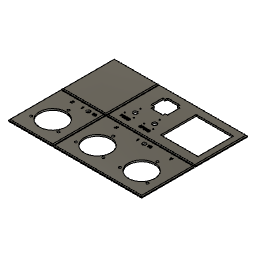
cnc3018_ctrl v79 (Autodesk Fusion 360 design; units mm, degrees)
Autodesk Fusion 360 part; units mm, degrees
sketch "panel" plane through (0, 0, 0) normal (0, 0, 1) x (1, 0, 0)
  line L0 (0, 0) -> (71, 0)
  line L1 (71, 0) -> (71, 84.5)
  line L2 (71, 84.5) -> (0, 84.5)
  line L3 (0, 84.5) -> (0, 0)
  line L4 (35.5, 84.5) -> (35.5, 0) construction
  circle A0 centre (35.5, 35.5) radius 30.5 construction
  line L5 (35.5, 66) -> (71, 66) construction
  line L6 (46.5, 79.5) -> (59.5, 79.5) construction
  line L7 (59.5, 79.5) -> (59.5, 71) construction
  line L8 (59.5, 71) -> (46.5, 71) construction
  line L9 (46.5, 71) -> (46.5, 79.5) construction
  line L10 (46.5, 79.5) -> (59.5, 71) construction
  circle A1 centre (53, 75.25) radius 3
  line L11 (66, 79.5) -> (40, 79.5) construction
  line L12 (40, 79.5) -> (40, 71) construction
  line L13 (40, 71) -> (66, 71) construction
  line L14 (66, 71) -> (66, 79.5) construction
  line L15 (66, 79.5) -> (40, 71) construction
  line L16 (40, 79.5) -> (66, 71) construction
  line L17 (40, 71) -> (46.5, 71) construction
  line L18 (46.5, 71) -> (46.5, 79.5) construction
  line L19 (46.5, 79.5) -> (40, 79.5) construction
  line L20 (40, 79.5) -> (40, 71) construction
  line L21 (59.5, 71) -> (66, 71) construction
  line L22 (66, 71) -> (66, 79.5) construction
  line L23 (66, 79.5) -> (59.5, 79.5) construction
  line L24 (59.5, 79.5) -> (59.5, 71) construction
  line L25 (24, 79.5) -> (30.5, 79.5) construction
  line L26 (30.5, 79.5) -> (30.5, 71) construction
  line L27 (30.5, 71) -> (24, 71) construction
  line L28 (24, 71) -> (24, 79.5) construction
  line L29 (24, 71) -> (30.5, 71) construction
  line L30 (30.5, 71) -> (30.5, 79.5) construction
  line L31 (30.5, 79.5) -> (24, 79.5) construction
  line L32 (24, 79.5) -> (24, 71) construction
  circle A2 centre (35.5, 35.5) radius 21.25
  circle A3 centre (35.5, 60.9) radius 1.75
  circle A4 centre (13.503, 22.8) radius 1.75
  circle A5 centre (57.497, 22.8) radius 1.75
  line L33 (71, 0) -> (213, 0)
  line L34 (213, 0) -> (213, 84.5)
  line L35 (213, 84.5) -> (71, 84.5)
  line L36 (71, 84.5) -> (71, 0)
  line L37 (35.5, 35.5) -> (213, 35.5) construction
  line L38 (53, 75.25) -> (213, 75.25) construction
  circle A6 centre (106.5, 35.5) radius 21.25
  circle A7 centre (106.5, 35.5) radius 30.5 construction
  line L39 (106.5, 35.5) -> (106.5, 84.5) construction
  circle A8 centre (106.5, 60.9) radius 1.75
  line L40 (35.5, 60.9) -> (213, 60.9) construction
  line L41 (35.5, 14.25) -> (213, 14.25) construction
  line L42 (35.5, 5) -> (213, 5) construction
  circle A9 centre (84.503, 22.8) radius 1.75
  circle A10 centre (128.497, 22.8) radius 1.75
  circle A11 centre (177.5, 35.5) radius 21.25
  circle A12 centre (177.5, 35.5) radius 30.5 construction
  line L43 (177.5, 35.5) -> (177.5, 84.5) construction
  circle A13 centre (177.5, 60.9) radius 1.75
  circle A14 centre (155.503, 22.8) radius 1.75
  circle A15 centre (199.497, 22.8) radius 1.75
  line L44 (142, 84.5) -> (142, 0) construction
  line L45 (148.5, 71) -> (135.5, 71) construction
  line L46 (135.5, 71) -> (135.5, 79.5) construction
  line L47 (135.5, 79.5) -> (148.5, 79.5) construction
  line L48 (148.5, 79.5) -> (148.5, 71) construction
  line L49 (148.5, 71) -> (135.5, 79.5) construction
  line L50 (135.5, 71) -> (148.5, 79.5) construction
  line L51 (155, 71) -> (129, 71) construction
  line L52 (129, 71) -> (129, 79.5) construction
  line L53 (129, 79.5) -> (155, 79.5) construction
  line L54 (155, 79.5) -> (155, 71) construction
  line L55 (155, 71) -> (129, 79.5) construction
  line L56 (129, 71) -> (155, 79.5) construction
  circle A16 centre (142, 75.25) radius 3
  line L57 (40, 71) -> (46.5, 71) construction
  line L58 (46.5, 71) -> (46.5, 79.5) construction
  line L59 (46.5, 79.5) -> (40, 79.5) construction
  line L60 (40, 79.5) -> (40, 71) construction
  line L61 (129, 71) -> (135.5, 71) construction
  line L62 (135.5, 71) -> (135.5, 79.5) construction
  line L63 (135.5, 79.5) -> (129, 79.5) construction
  line L64 (129, 79.5) -> (129, 71) construction
  line L65 (148.5, 71) -> (155, 71) construction
  line L66 (155, 71) -> (155, 79.5) construction
  line L67 (155, 79.5) -> (148.5, 79.5) construction
  line L68 (148.5, 79.5) -> (148.5, 71) construction
  line L69 (101.5, 79.5) -> (95, 79.5) construction
  line L70 (95, 79.5) -> (95, 71) construction
  line L71 (95, 71) -> (101.5, 71) construction
  line L72 (101.5, 71) -> (101.5, 79.5) construction
  line L73 (101.5, 79.5) -> (95, 71) construction
  line L74 (95, 79.5) -> (101.5, 71) construction
  line L75 (95, 71) -> (101.5, 71) construction
  line L76 (101.5, 71) -> (101.5, 79.5) construction
  line L77 (101.5, 79.5) -> (95, 79.5) construction
  line L78 (95, 79.5) -> (95, 71) construction
  line L79 (189, 79.5) -> (182.5, 79.5) construction
  line L80 (182.5, 79.5) -> (182.5, 71) construction
  line L81 (182.5, 71) -> (189, 71) construction
  line L82 (189, 71) -> (189, 79.5) construction
  line L83 (189, 79.5) -> (182.5, 71) construction
  line L84 (182.5, 79.5) -> (189, 71) construction
  line L85 (182.5, 71) -> (189, 71) construction
  line L86 (189, 71) -> (189, 79.5) construction
  line L87 (189, 79.5) -> (182.5, 79.5) construction
  line L88 (182.5, 79.5) -> (182.5, 71) construction
  line L89 (0, 84.5) -> (213, 84.5)
  line L90 (213, 84.5) -> (213, 169)
  line L91 (213, 169) -> (0, 169)
  line L92 (0, 169) -> (0, 84.5)
  line L93 (143, 156.5) -> (203, 156.5)
  line L94 (203, 156.5) -> (203, 99.5)
  line L95 (203, 99.5) -> (143, 99.5)
  line L96 (143, 99.5) -> (143, 156.5)
  line L97 (93.25, 156.5) -> (120.75, 156.5)
  line L98 (120.75, 156.5) -> (120.75, 129)
  line L99 (120.75, 129) -> (93.25, 129)
  line L100 (93.25, 129) -> (93.25, 156.5)
  line L101 (93.25, 156.5) -> (97.05, 156.5)
  line L102 (97.05, 156.5) -> (97.05, 152.7)
  line L103 (97.05, 152.7) -> (93.25, 152.7)
  line L104 (93.25, 152.7) -> (93.25, 156.5)
  line L105 (120.75, 156.5) -> (116.95, 156.5)
  line L106 (116.95, 156.5) -> (116.95, 152.7)
  line L107 (116.95, 152.7) -> (120.75, 152.7)
  line L108 (120.75, 152.7) -> (120.75, 156.5)
  line L109 (93.25, 129) -> (98.25, 129)
  line L110 (98.25, 129) -> (98.25, 134)
  line L111 (98.25, 134) -> (93.25, 134)
  line L112 (93.25, 134) -> (93.25, 129)
  line L113 (120.75, 129) -> (116.95, 129)
  line L114 (116.95, 129) -> (116.95, 132.8)
  line L115 (116.95, 132.8) -> (120.75, 132.8)
  line L116 (120.75, 132.8) -> (120.75, 129)
  line L117 (71, 84.5) -> (71, 169)
  line L118 (76, 124) -> (138, 124) construction
  line L119 (138, 124) -> (138, 89.5) construction
  line L120 (138, 89.5) -> (76, 89.5) construction
  line L121 (76, 89.5) -> (76, 124) construction
  circle A17 centre (91.5, 110.25) radius 3.5
  circle A18 centre (91.5, 110.25) radius 10.5 construction
  line L122 (81, 120.75) -> (102, 120.75) construction
  line L123 (102, 120.75) -> (102, 92.75) construction
  line L124 (102, 92.75) -> (81, 92.75) construction
  line L125 (81, 92.75) -> (81, 120.75) construction
  line L126 (91.5, 110.25) -> (91.5, 120.75) construction
  line L127 (81, 92.75) -> (102, 92.75) construction
  line L128 (102, 92.75) -> (102, 99.75) construction
  line L129 (102, 99.75) -> (81, 99.75) construction
  line L130 (81, 99.75) -> (81, 92.75) construction
  line L131 (81, 92.75) -> (102, 92.75) construction
  line L132 (102, 92.75) -> (102, 99.75) construction
  line L133 (102, 99.75) -> (81, 99.75) construction
  line L134 (81, 99.75) -> (81, 92.75) construction
  line L135 (76, 124) -> (107, 124) construction
  line L136 (107, 124) -> (76, 89.5) construction
  line L137 (81, 120.75) -> (102, 92.75) construction
  line L138 (91.5, 110.25) -> (98.9246, 102.8254) construction
  line L139 (91.5, 110.25) -> (84.0754, 102.8254) construction
  circle A19 centre (91.5, 120.75) radius 0.875
  circle A20 centre (84.0754, 102.8254) radius 0.875
  circle A21 centre (98.9246, 102.8254) radius 0.875
  line L140 (107, 124) -> (138, 89.5) construction
  line L141 (143, 156.5) -> (71, 156.5) construction
  line L142 (107, 124) -> (107, 89.5) construction
  line L143 (133, 92.75) -> (112, 92.75) construction
  line L144 (112, 120.75) -> (133, 120.75) construction
  line L145 (112, 92.75) -> (133, 92.75) construction
  line L146 (112, 120.75) -> (133, 92.75) construction
  circle A22 centre (122.5, 110.25) radius 10.5 construction
  line L147 (122.5, 110.25) -> (129.9246, 102.8254) construction
  circle A23 centre (129.9246, 102.8254) radius 0.875
  line L148 (122.5, 110.25) -> (122.5, 120.75) construction
  line L149 (133, 120.75) -> (133, 92.75) construction
  line L150 (122.5, 110.25) -> (115.0754, 102.8254) construction
  line L151 (133, 99.75) -> (112, 99.75) construction
  line L152 (133, 92.75) -> (133, 99.75) construction
  circle A24 centre (122.5, 120.75) radius 0.875
  circle A25 centre (115.0754, 102.8254) radius 0.875
  line L153 (112, 99.75) -> (112, 92.75) construction
  line L154 (112, 92.75) -> (112, 120.75) construction
  circle A26 centre (122.5, 110.25) radius 3.5
  line L155 (112, 92.75) -> (133, 92.75) construction
  line L156 (133, 92.75) -> (133, 99.75) construction
  line L157 (133, 99.75) -> (112, 99.75) construction
  line L158 (112, 99.75) -> (112, 92.75) construction
  point P0 (53, 75.25)
  point P1 (142, 75.25)
  point P2 (142, 75.25)
  point P3 (98.25, 75.25)
  point P4 (185.75, 75.25)
  point P5 (107, 156.5)
  point P6 (91.5, 106.75)
  point P7 (122.5, 106.75)
  dimension "d120" = 61
  dimension "d122" = 71
  dimension "d123" = 5
  dimension "d124" = 13
  dimension "d125" = 8.5
  dimension "d126" = 6
  dimension "d127" = 26
  dimension "d128" = 8.5
  dimension "d129" = 4
  dimension "d130" = 4
  dimension "d131" = 5
  dimension "d132" = 5
  dimension "d133" = 5
  dimension "d134" = 6.5
  dimension "d135" = 8.5
  dimension "d136" = 5
  dimension "d137" = 5
  dimension "d138" = 4
  dimension "d139" = 42.5
  dimension "d140" = 3.5
  dimension "d141" = 25.4
  dimension "d144" = 360
  dimension "d145" = 142
  dimension "d149" = 5
  dimension "d150" = 3.5
  dimension "d153" = 360
  dimension "d154" = 5
  dimension "d155" = 3.5
  dimension "d157" = 360
  dimension "d158" = 13
  dimension "d159" = 8.5
  dimension "d160" = 26
  dimension "d161" = 8.5
  dimension "d162" = 6
  dimension "d163" = 4
  dimension "d164" = 4
  dimension "d165" = 4
  dimension "d166" = 6.5
  dimension "d167" = 8.5
  dimension "d168" = 5
  dimension "d169" = 4
  dimension "d170" = 6.5
  dimension "d171" = 8.5
  dimension "d172" = 5
  dimension "d173" = 4
  dimension "d184" = 84.5
  dimension "d185" = 84.5
  dimension "d186" = 60
  dimension "d187" = 57
  dimension "d188" = 10
  dimension "d189" = 15
  dimension "d190" = 27.5
  dimension "d191" = 27.5
  dimension "d192" = 3.8
  dimension "d193" = 3.8
  dimension "d194" = 3.8
  dimension "d195" = 3.8
  dimension "d196" = 5
  dimension "d197" = 5
  dimension "d198" = 3.8
  dimension "d199" = 3.8
  dimension "d200" = 12.5
  dimension "d201" = 12.5
  dimension "d203" = 5
  dimension "d204" = 5
  dimension "d205" = 5
  dimension "d206" = 5
  dimension "d207" = 7
  dimension "d208" = 21
  dimension "d209" = 21
  dimension "d212" = 28
  dimension "d213" = 4
  dimension "d214" = 135
  dimension "d215" = 135
  dimension "d216" = 1.75
  dimension "d217" = 1.75
  dimension "d218" = 1.75
  dimension "d221" = 31
  dimension "d222" = 0
  dimension "d223" = 4
  text T0 "1" font "Arial" height 4 align centre middle in box 6.5 x 8.5 at (40, 71) x (1, 0) y (0, 1) spacing 1
  text T1 "10" font "Arial" height 4 align centre middle in box 6.5 x 8.5 at (59.5, 71) x (1, 0) y (0, 1) spacing 1
  text T2 "Z" font "Arial" height 4 align centre middle in box 6.5 x 8.5 at (24, 71) x (1, 0) y (0, 1) spacing 1
  text T3 "1" font "Arial" height 4 align centre middle in box 6.5 x 8.5 at (129, 71) x (1, 0) y (0, 1) spacing 1
  text T4 "10" font "Arial" height 4 align centre middle in box 6.5 x 8.5 at (148.5, 71) x (1, 0) y (0, 1) spacing 1
  text T5 "X" font "Arial" height 4 align centre middle in box 6.5 x 8.5 at (95, 71) x (1, 0) y (0, 1) spacing 1
  text T6 "Y" font "Arial" height 4 align centre middle in box 6.5 x 8.5 at (182.5, 71) x (1, 0) y (0, 1) spacing 1
  text T7 "FEED" font "Arial" height 4 align centre middle in box 21 x 7 at (81, 92.75) x (1, 0) y (0, 1) spacing 1
  text T8 "SPIND" font "Arial" height 4 align centre middle in box 21 x 7 at (112, 92.75) x (1, 0) y (0, 1) spacing 1
  constraint horizontal L0
  constraint vertical L1
  constraint horizontal L2
  constraint vertical L3
  constraint coincident L0.start L3.end
  constraint midpoint L2 L4.start
  constraint midpoint L0 L4.end
  constraint coincident A0 L5.start
  constraint coincident L4 L5.start
  constraint coincident L1 L5.end
  constraint tangent A0 L5
  constraint perpendicular L1 L5
  constraint horizontal L6
  constraint vertical L7
  constraint horizontal L8
  constraint vertical L9
  constraint coincident L10 P0
  constraint horizontal L11
  constraint perpendicular L11 L12
  constraint parallel L11 L13
  constraint parallel L12 L14
  constraint coincident L15 P0
  constraint coincident L16 P0
  constraint coincident P0 A1.centre
  constraint midpoint L10 P0
  constraint coincident L8.end
  constraint coincident L11.end
  constraint coincident L13.end
  constraint coincident L6.end
  constraint horizontal L25
  constraint vertical L26
  constraint horizontal L27
  constraint vertical L28
  constraint coincident L26.end
  constraint coincident L25.start
  constraint concentric A0 A2
  constraint coincident L4 A3.centre
  constraint horizontal L33
  constraint vertical L34
  constraint horizontal L35
  constraint vertical L36
  constraint coincident A0.centre A2.centre
  constraint coincident L34 L37.end
  constraint perpendicular L34 L37
  constraint coincident L34 L38.end
  constraint perpendicular L34 L38
  constraint coincident L37 A6.centre
  constraint concentric A6 A7
  constraint coincident A6.centre A7.centre
  constraint coincident L35 L39.end
  constraint perpendicular L35 L39
  constraint coincident L39 A8.centre
  constraint coincident A3.centre L40.start
  constraint coincident L34 L40.end
  constraint perpendicular L34 L40
  constraint coincident A8.centre L40
  constraint coincident A2 L41.start
  constraint coincident L4 L41.start
  constraint coincident L34 L41.end
  constraint tangent A2 L41
  constraint coincident A0 L42.start
  constraint coincident L4 L42.start
  constraint coincident L34 L42.end
  constraint tangent A0 L42
  constraint tangent A7 L42
  constraint tangent A6 L41
  constraint coincident L37 A11.centre
  constraint tangent L41 A11
  constraint concentric A11 A12
  constraint tangent L42 A12
  constraint coincident A11.centre A12.centre
  constraint coincident L35 L43.end
  constraint perpendicular L35 L43
  constraint coincident L43 A13.centre
  constraint coincident L40 A13.centre
  constraint midpoint L35 L44.start
  constraint midpoint L33 L44.end
  constraint horizontal L45
  constraint perpendicular L45 L46
  constraint parallel L45 L47
  constraint parallel L46 L48
  constraint coincident L49 P2
  constraint coincident L50 P2
  constraint coincident L44 P2
  constraint coincident L38 P2
  constraint horizontal L51
  constraint perpendicular L51 L52
  constraint parallel L51 L53
  constraint parallel L52 L54
  constraint coincident L55 P2
  constraint coincident L56 P2
  constraint coincident P2 P1
  constraint coincident L45.end
  constraint coincident L52.end
  constraint coincident L51.start
  constraint coincident L47.end
  constraint horizontal L69
  constraint perpendicular L69 L70
  constraint parallel L69 L71
  constraint parallel L70 L72
  constraint coincident L73 P3
  constraint coincident L74 P3
  constraint coincident L38 P3
  constraint coincident L71.end
  constraint coincident L69.end
  constraint horizontal L79
  constraint perpendicular L79 L80
  constraint parallel L79 L81
  constraint parallel L80 L82
  constraint coincident L83 P4
  constraint coincident L84 P4
  constraint coincident L38 P4
  constraint coincident L81.end
  constraint coincident L79.end
  constraint horizontal L89
  constraint vertical L90
  constraint horizontal L91
  constraint vertical L92
  constraint horizontal L93
  constraint vertical L94
  constraint horizontal L95
  constraint vertical L96
  constraint horizontal L97
  constraint vertical L98
  constraint horizontal L99
  constraint vertical L100
  constraint horizontal L101
  constraint vertical L102
  constraint horizontal L103
  constraint vertical L104
  constraint horizontal L105
  constraint vertical L106
  constraint horizontal L107
  constraint vertical L108
  constraint horizontal L109
  constraint vertical L110
  constraint horizontal L111
  constraint vertical L112
  constraint horizontal L113
  constraint vertical L114
  constraint horizontal L115
  constraint vertical L116
  constraint midpoint L97 P5
  constraint coincident L91 L117.end
  constraint perpendicular L91 L117
  constraint horizontal L118
  constraint vertical L119
  constraint horizontal L120
  constraint vertical L121
  constraint concentric A17 A18
  constraint horizontal L122
  constraint vertical L123
  constraint horizontal L124
  constraint vertical L125
  constraint tangent A18 L122
  constraint tangent A18 L125
  constraint coincident A17.centre A18.centre
  constraint midpoint L122 L126.end
  constraint horizontal L127
  constraint vertical L128
  constraint horizontal L129
  constraint vertical L130
  constraint coincident L123 L128.end
  constraint tangent A18 L129
  constraint coincident L123.end
  constraint coincident L129.end
  constraint midpoint L118 L135.end
  constraint coincident L137 P6
  constraint midpoint L137 P6
  constraint midpoint L136 P6
  constraint coincident A18 L138.end
  constraint coincident A18 L139.end
  constraint coincident L126.end A19.centre
  constraint coincident L139.end A20.centre
  constraint coincident L138.end A21.centre
  constraint coincident L117 L141.end
  constraint perpendicular L117 L141
  constraint midpoint P5 L141
  constraint midpoint L120 L142.end
  constraint coincident L143.start
  constraint coincident L151.end
  measures "d120" diameter of A0
  measures "d122" distance of L0.start L0.end
  measures "d123" distance of L0 A0
  measures "d124" distance of L6.start L6.end
  measures "d125" distance of L6.end L7.end
  measures "d126" diameter of A1
  measures "d127" distance of L12.end L13.end
  measures "d128" distance of L11.end L12.end
  measures "d131" distance of L2 L11
  measures "d132" distance of L5 L13
  measures "d133" distance of L1 L14
  measures "d134" distance of L25.start L25.end
  measures "d135" distance of L25.start L27.end
  measures "d136" distance of L4 L26
  measures "d137" distance of A0 L27
  measures "d139" diameter of A2
  measures "d140" diameter of A3
  measures "d141" distance of A0.centre A3.centre
  measures "d145" distance of L0.end L33.end
  measures "d149" distance of L1 A7
  measures "d150" diameter of A8
  measures "d154" distance of L34 A12
  measures "d155" diameter of A13
  measures "d158" distance of L46.end L47.end
  measures "d159" distance of L45.end L46.end
  measures "d160" distance of L52.end L53.end
  measures "d161" distance of L51.end L52.end
  measures "d162" diameter of A16
  measures "d166" distance of L70.end L71.end
  measures "d167" distance of L69.end L70.end
  measures "d168" distance of L39 L72
  measures "d170" distance of L80.end L81.end
  measures "d171" distance of L79.end L80.end
  measures "d172" distance of L43 L80
  measures "d184" distance of L0.start L2.end
  measures "d185" distance of L2.end L91.end
  measures "d186" distance of L93.start L93.end
  measures "d187" distance of L93.start L95.end
  measures "d188" distance of L90 L94
  measures "d189" distance of L89 L95
  measures "d190" distance of L97.start L97.end
  measures "d191" distance of L97.start L99.end
  measures "d192" distance of L97.start L101.end
  measures "d193" distance of L97.start L103.end
  measures "d194" distance of L97.end L105.end
  measures "d195" distance of L97.end L107.end
  measures "d196" distance of L99.end L109.end
  measures "d197" distance of L99.end L111.end
  measures "d198" distance of L98.end L113.end
  measures "d199" distance of L98.end L115.end
  measures "d200" distance of L91 L93
  measures "d201" distance of L91 L97
  measures "d203" distance of L89 L120
  measures "d204" distance of L117 L121
  measures "d205" distance of L99 L118
  measures "d206" distance of L96 L119
  measures "d207" diameter of A17
  measures "d208" diameter of A18
  measures "d209" distance of L122.start L122.end
  measures "d212" distance of L122.start L124.end
  measures "d214" angle of L126 L138
  measures "d215" angle of L126 L139
  measures "d216" diameter of A19
  measures "d217" diameter of A20
  measures "d218" diameter of A21
extrude "Extrude10" add sketch "panel" along normal blind 2.5 contours L0 L1 L2 L3 L36 L89 makes body 1
extrude "Extrude11" add sketch "panel" along normal blind 2.5 separate body contours L1 L33 L34 L35 L36 L89 makes body 2
move_body "Move5" bodies 2 to x (1, 0, 0) y (0, 1, 0) z (0, 0, 1) at (1, 0, 0)
extrude "Extrude13" add sketch "panel" along normal blind 2.5 separate body contours L35 L89 L90 L91 L117 | L97 L100 L101 L102 L103 L104 | L97 L98 L105 L106 L107 L108 | L99 L100 L109 L110 L111 L112 | L98 L99 L113 L114 L115 L116 | A19 | A20 | A21 | A23 | A24 | A25 makes body 3
move_body "Move6" bodies 3 to x (1, 0, 0) y (0, 1, 0) z (0, 0, 1) at (1, 1, 0)
extrude "Extrude14" add sketch "panel" along normal blind 2.5 separate body contours L2 L89 L91 L92 L117 makes body 4
move_body "Move7" bodies 4 to x (1, 0, 0) y (0, 1, 0) z (0, 0, 1) at (0, 1, 0)
extrude "Extrude12" add sketch "panel" sketch "panel" along normal blind 0.5 contours A19 | A20 | A21 | A23 | A24 | A25 of sketch 2 text T2 T0 T1 T5 T3 T4 T6 T7 T8 start surface through (1, 0, 2.5) normal (0, 0, 1) bodies 1 2 3
fillet "Fillet6" radius 1.25 16 edges at (35.5, 84.5, 2.5) (0, 42.25, 2.5) (35.5, 0, 2.5) (71, 42.25, 2.5) (143, 84.5, 2.5) (72, 42.25, 2.5) (143, 0, 2.5) (214, 42.25, 2.5) (143, 170, 2.5) (214, 127.75, 2.5) (72, 127.75, 2.5) (143, 85.5, 2.5) (71, 127.75, 2.5) (35.5, 170, 2.5) (0, 127.75, 2.5) (35.5, 85.5, 2.5) on bodies 1 2 3 4
equation "enc_bolt = 3.5 mm"
equation "enc_hole = 42.5 mm"
equation "switch_w = 13 mm"
equation "switch_l = 8.5 mm"
equation "switch_hole = 6 mm"
equation "panel_angle = 35 deg"
equation "enc_outside = 61 mm"
equation "d120 = enc_outside"
equation "enc_space = 5 mm"
equation "d122 = enc_outside + 2 * enc_space"
equation "d123 = enc_space"
equation "d124 = switch_w"
equation "d125 = switch_l"
equation "d126 = switch_hole"
equation "d127 = 2 * switch_w"
equation "d128 = switch_l"
equation "d131 = enc_space"
equation "d132 = enc_space"
equation "d133 = enc_space"
equation "d134 = switch_w / 2"
equation "d135 = switch_l"
equation "d136 = enc_space"
equation "d137 = enc_space"
equation "d139 = enc_hole"
equation "d140 = enc_bolt"
equation "d141 = enc_bolt_r"
equation "enc_bolt_r = ( 50.8 / 2 ) * 1 mm"
equation "d145 = 2 * d122"
equation "d149 = enc_space"
equation "d150 = enc_bolt"
equation "d154 = enc_space"
equation "d155 = enc_bolt"
equation "d158 = switch_w"
equation "d159 = switch_l"
equation "d160 = 2 * switch_w"
equation "d161 = switch_l"
equation "d162 = switch_hole"
equation "d166 = switch_w / 2"
equation "d167 = switch_l"
equation "d168 = enc_space"
equation "d170 = switch_w / 2"
equation "d171 = switch_l"
equation "d172 = enc_space"
equation "d174 = panel_th"
equation "panel_th = 2.5 mm"
equation "d177 = panel_th"
equation "d185 = d184"
equation "d188 = 2 * enc_space"
equation "d189 = 3 * enc_space"
equation "d192 = d193"
equation "d194 = d193"
equation "d195 = d193"
equation "d198 = d193"
equation "d199 = d193"
equation "d201 = d200"
equation "resistor_hole = 7 mm"
equation "d203 = enc_space"
equation "d204 = enc_space"
equation "d205 = enc_space"
equation "d206 = enc_space"
equation "d207 = resistor_hole"
equation "d208 = 3 * resistor_hole"
equation "d209 = 3 * resistor_hole"
equation "d212 = 4 * resistor_hole"
equation "d214 = ( 270 / 2 ) * 1 deg"
equation "d215 = ( 270 / 2 ) * 1 deg"
equation "d216 = enc_bolt / 2"
equation "d217 = enc_bolt / 2"
equation "d218 = enc_bolt / 2"
equation "d224 = panel_th"
equation "d227 = panel_th / 2"
equation "d228 = panel_th"
named bodies: "xy", "kbd"
